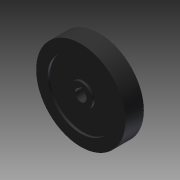
# Autodesk Inventor part: wheel
Saved by Autodesk Inventor 2011 SP1 (Build 150282100, 282)
## iProperties
Created: 2012-01-14
Part Number: wheel
Document SubType Name: Modeling
Designer: Christopher
Density: 1 g/cm^3
Author: Christopher
Autodesk Inventor part; units mm, degrees
ref_plane "YZ Plane" through (0, 0, 0) normal (1, 0, 0) x (0, 1, 0)
ref_plane "XZ Plane" through (0, 0, 0) normal (0, 1, 0) x (-1, 0, 0)
ref_plane "XY Plane" through (0, 0, 0) normal (0, 0, 1) x (1, 0, 0)
sketch "Sketch1" plane through (0, 0, 0) normal (0, 0, 1) x (1, 0, 0)
  circle A0 centre (0, 0) radius 49.2125
  circle A1 centre (0, 0) radius 6.35
  circle A2 centre (0, 0) radius 36.5125
  circle A3 centre (0, 0) radius 12.7
  line L0 (-1.5875, 7.9375) -> (1.5875, 7.9375)
  line L1 (1.5875, 7.9375) -> (1.5875, 6.1484)
  line L2 (1.5875, 6.1484) -> (-1.5875, 6.1484)
  line L3 (-1.5875, 6.1484) -> (-1.5875, 7.9375)
  point P0 (0, 6.1484)
  dimension "d1" = 12.7
  dimension "d0" = 98.425
  dimension "d2" = 12.7
  dimension "d3" = 25.4
  dimension "d10" = 7.9375
  dimension "d11" = 3.175
  constraints: 8 end point, 4 coincident, 3 centre point, 2 parallel, 1 horizontal, 1 midpoint, 1 perpendicular, 1 vertical alignment, 3 other
  measures "d0" diameter of A0
  measures "d2" radial gap between concentric circles of A0 A2
  measures "d3" diameter of A3
  measures "d10" distance from line of point (0, 0) L0
  measures "d11" distance between parallel lines of L3 L1
extrude "Extrusion1" add sketch "Sketch1" along normal mid plane 20.32 contours A0
extrude "Extrusion2" add sketch "Sketch1" along normal mid plane 15.24 contours A2
extrude "Extrusion3" add sketch "Sketch1" along normal mid plane 20.32 contours L2 A1 | A1 L3 L0 L1 | A3 picked at (-0.1781, 6.2081)
extrude "Extrusion4" cut sketch "Sketch1" along normal mid plane 25.4 contours L2 A1 | A1 L3 L0 L1 picked at (-0.1781, 6.2081)
body "Solid1"
